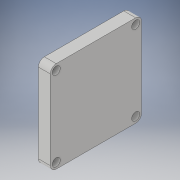
# Autodesk Inventor part: HGLRC Micro 13A 4in1 BLHeli_S
Saved by Autodesk Inventor 2018 (Build 220112000, 112)
## iProperties
Created: 2018-01-27
Part Number: HGLRC Micro 13A 4in1 BLHeli_S
Material: Všeobecné
Document SubType Name: Modeling
Designer: Kuba
Density: 1 g/cm^3
Appearance: Výchozí
Author: Kuba
Autodesk Inventor part; units mm, degrees
ref_plane "YZ Plane" through (0, 0, 0) normal (1, 0, 0) x (0, 1, 0)
ref_plane "XZ Plane" through (0, 0, 0) normal (0, 1, 0) x (-1, 0, 0)
ref_plane "XY Plane" through (0, 0, 0) normal (0, 0, 1) x (1, 0, 0)
sketch "Náčrt1" plane through (0, 0, 0) normal (1, 0, 0) x (0, 1, 0)
  line L0 (1.5, 0) -> (21.5, 0)
  line L1 (23, -1.5) -> (23, -21.5)
  line L2 (21.5, -23) -> (1.5, -23)
  line L3 (0, -21.5) -> (0, -1.5)
  arc A0 (23, -1.5) -> (21.5, 0) centre (21.5, -1.5) ccw
  arc A1 (21.5, -23) -> (23, -21.5) centre (21.5, -21.5) ccw
  arc A2 (0, -21.5) -> (1.5, -23) centre (1.5, -21.5) ccw
  arc A3 (1.5, 0) -> (0, -1.5) centre (1.5, -1.5) ccw
  circle A4 centre (21.5, -1.5) radius 1
  circle A5 centre (1.5, -21.5) radius 1
  circle A6 centre (1.5, -1.5) radius 1
  circle A7 centre (21.5, -21.5) radius 1
  point P0 (0, 0)
  point P1 (23, 0)
  point P2 (0, -23)
  dimension "d0" = 23
  dimension "d1" = 23
  dimension "d2" = 1.5
  dimension "d3" = 1.5
  dimension "d4" = 2
  dimension "d5" = 2
  dimension "d6" = 2
  dimension "d7" = 2
  constraints: 8 centre point, 8 end point, 8 point on circle, 8 tangent, 7 coincident, 6 point on line, 2 equal radius, 2 parallel, 1 horizontal, 1 perpendicular
  measures "d0" distance of point (0, 0) point (23, 0)
  measures "d1" distance of point (0, -23) point (0, 0)
  measures "d2" radius of A0
  measures "d3" radius of A3
  measures "d4" diameter of A4
  measures "d5" diameter of A5
  measures "d6" diameter of A6
  measures "d7" diameter of A7
extrude "Vysunutí1" add sketch "Náčrt1" along normal blind 3
equation "\"d1\" = d0"
